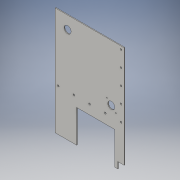
# Autodesk Inventor part: 1073-2017 Shooter Outside Plate Right
Saved by Autodesk Inventor 2016 (Build 200138000, 138)
## iProperties
Created: 2017-01-29
Part Number: 1073-2017 Shooter Outside Plate Right
Material: Generic
Document SubType Name: Modeling
Designer: rasmussenf
Density: 1 g/cm^3
Appearance: Default
Author: rasmussenf
Autodesk Inventor part; units mm, degrees
ref_plane "YZ Plane" through (0, 0, 0) normal (1, 0, 0) x (0, 1, 0)
ref_plane "XZ Plane" through (0, 0, 0) normal (0, 1, 0) x (-1, 0, 0)
ref_plane "XY Plane" through (0, 0, 0) normal (0, 0, 1) x (1, 0, 0)
sketch "Sketch1" plane through (0, 0, 0) normal (0, 0, 1) x (1, 0, 0)
  line L0 (279.4, 279.4) -> (0, 279.4)
  line L1 (0, 279.4) -> (0, 0)
  circle A0 centre (50.8, 228.6) radius 14.2875
  circle A1 centre (50.8, 228.6) radius 250.0376 construction
  circle A2 centre (227.6033, 51.7967) radius 14.2875
  line L2 (50.8, 228.6) -> (279.4, 0) construction
  line L3 (279.4, 279.4) -> (279.4, -131.826)
  line L4 (279.4, -131.826) -> (253.746, -131.826)
  line L5 (253.746, -131.826) -> (253.746, -157.48)
  line L6 (253.746, -157.48) -> (241.3, -157.48)
  line L7 (241.3, -157.48) -> (241.3, -25.4)
  line L8 (241.3, -25.4) -> (87.1728, -25.4)
  line L9 (87.1728, -25.4) -> (87.1728, -157.48)
  line L10 (87.1728, -157.48) -> (0, -157.48)
  line L11 (0, -157.48) -> (0, 0)
  dimension "d5" = 500.0752
  dimension "d0" = 279.4
  dimension "d1" = 279.4
  dimension "d2" = 28.575
  dimension "d6" = 28.575
  dimension "d36" = 411.226
  dimension "d37" = 25.654
  dimension "d38" = 25.654
  dimension "d39" = 12.446
  dimension "d40" = 132.08
  dimension "d41" = 154.1272
  constraints: 24 end point, 6 perpendicular, 3 point on line, 2 centre point, 1 coincident, 1 parallel, 1 vertical, 3 other
  measures "d0" distance of L0.start L0.end
  measures "d1" distance of L2.end L0.start
  measures "d2" diameter of A0
  measures "d6" diameter of A2
  measures "d36" distance of L0.start L3.end
  measures "d37" distance of L3.end L4.end
  measures "d38" distance of L4.end L5.end
  measures "d39" distance of L5.end L6.end
  measures "d40" distance of L6.end L7.end
  measures "d41" distance of L7.end L8.end
extrude "Extrusion1" add sketch "Sketch1" along normal blind 3.175
sketch "Sketch2" plane through (0, 0, 3.175) normal (0, 0, 1) x (1, 0, 0)
  circle A0 centre (266.7, 12.7) radius 3.5687
  line L0 (0, 0) -> (279.4, 0) projected
  line L1 (279.4, 0) -> (279.4, 279.4) projected
  circle A1 centre (266.7, 76.2) radius 3.5687
  circle A2 centre (266.7, 139.7) radius 3.5687
  circle A3 centre (266.7, 203.2) radius 3.5687
  circle A4 centre (266.7, 266.7) radius 3.5687
  circle A5 centre (203.2, 12.7) radius 3.5687
  circle A6 centre (139.7, 12.7) radius 3.5687
  circle A7 centre (76.2, 12.7) radius 3.5687
  circle A8 centre (12.7, 12.7) radius 3.5687
  dimension "d9" = 7.1374
  dimension "d10" = 12.7
  dimension "d11" = 12.7
  dimension "d14" = 63.5
  dimension "d24" = 63.5
  constraints: 9 centre point, 1 horizontal, 1 vertical, 16 other
  measures "d9" diameter of A0
  measures "d10" distance from line of L0 A0.centre
  measures "d11" distance from line of L1 A0.centre
  measures "d14" distance of A0.centre A1.centre
  measures "d24" distance of A0.centre A5.centre
extrude "Extrusion2" cut sketch "Sketch2" against normal blind 3.175
sketch "Sketch3" plane through (0, 0, 3.175) normal (0, 0, 1) x (1, 0, 0)
  circle A0 centre (227.6033, 51.7967) radius 14.195
  circle A1 centre (209.6428, 69.7572) radius 2.0193
  circle A2 centre (245.5638, 33.8362) radius 2.0193
  line L0 (206.6033, 58.9967) -> (206.6033, 44.5967)
  line L1 (206.6033, 44.5967) -> (205.3783, 43.3717)
  line L2 (205.3783, 43.3717) -> (205.3783, 37.7967)
  line L3 (205.3783, 37.7967) -> (211.6033, 37.7967)
  arc A3 (213.6033, 35.7967) -> (211.6033, 37.7967) centre (211.6033, 35.7967) ccw
  line L4 (213.6033, 35.7967) -> (213.6033, 30.7967)
  line L5 (213.6033, 30.7967) -> (247.6033, 30.7967)
  arc A4 (247.6033, 30.7967) -> (248.6033, 31.7967) centre (227.6033, 51.7967) ccw
  line L6 (248.6033, 31.7967) -> (248.6033, 33.5967)
  line L7 (248.6033, 33.5967) -> (249.8283, 34.8217)
  line L8 (249.8283, 34.8217) -> (249.8283, 43.3717)
  line L9 (249.8283, 43.3717) -> (248.6033, 44.5967)
  line L10 (248.6033, 44.5967) -> (248.6033, 58.9967)
  line L11 (248.6033, 58.9967) -> (249.8283, 60.2217)
  line L12 (249.8283, 60.2217) -> (249.8283, 65.7967)
  line L13 (249.8283, 65.7967) -> (243.6033, 65.7967)
  arc A5 (241.6033, 67.7967) -> (243.6033, 65.7967) centre (243.6033, 67.7967) ccw
  line L14 (241.6033, 67.7967) -> (241.6033, 72.7967)
  line L15 (241.6033, 72.7967) -> (207.6033, 72.7967)
  arc A6 (207.6033, 72.7967) -> (206.6033, 71.7967) centre (227.6033, 51.7967) ccw
  line L16 (206.6033, 71.7967) -> (206.6033, 69.9967)
  line L17 (206.6033, 69.9967) -> (205.3783, 68.7717)
  line L18 (205.3783, 68.7717) -> (205.3783, 60.2217)
  line L19 (205.3783, 60.2217) -> (206.6033, 58.9967)
  circle A7 centre (227.6033, 51.7967) radius 14.2875 projected
  point P0 (0, 0)
  dimension "d28" = 3.0395
  dimension "d29" = 4.2645
  dimension "d30" = 21
  dimension "d31" = 21
  dimension "d32" = 3.0395
  dimension "d33" = 4.2645
  constraints: 40 end point, 8 point on circle, 7 centre point, 1 concentric
  measures "d28" distance from line of L15 A1.centre
  measures "d29" distance from line of L18 A1.centre
  measures "d30" distance from line of L0 A0.centre
  measures "d31" distance from line of L15 A0.centre
  measures "d32" distance from line of L5 A2.centre
  measures "d33" distance from line of L8 A2.centre
extrude "Extrusion3" cut sketch "Sketch3" against normal blind 25.4 contours A1 | A2
body "Solid1"
